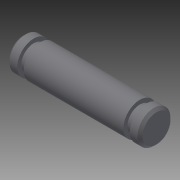
# Autodesk Inventor part: D-9769-clevis_pin
Saved by Autodesk Inventor 2014 (Build 180170000, 170)
## iProperties
Created: 2014-01-19
Part Number: D-9769-clevis_pin
Material: Steel
Catalog Web Link: www.cadenas.de
Description: Pivot Bracket for Original Line Cylinders - Clevis Pin-
Vendor: BIMBA
Document SubType Name: Standard Catalog Part
Designer: Michael
Manufacturer: BIMBA
Density: 7.85 g/cm^3
Appearance: Steel
Mass: 1.44762 g
Surface Area: 2.32572 cm^2
Volume: 0.18441 cm^3
Category: PARTsolutions
Company: BIMBA
PSOL_IDENT_0: {$CADENAS_DATA\23d-libs\bimba\bimba\bimba_imperial\bimba_full_line\original_line_cylinders\accessori
PSOL_IDENT_1: es\clevis_pin.prj},224 {VTYP=3D},{NB=D-9769-clevis_pin},{LINA=D-9769-clevis_pin},{NN=Pivot Bracket f
PSOL_IDENT_2: or Original Line Cylinders - Clevis Pin},{DATE=06.12.2011 07:07:55},{GEOMDATE=06.12.2011 00:00:00},{
PSOL_IDENT_3: VERSION=},{LINEID=30},{LINESUBID=-1},{WBVAR=}  {NB=D-9769-clevis_pin},{LINA=D-9769-clevis_pin},{KT=D
PSOL_IDENT_4: UMMY},{PN=D-9769},{MAT=Zinc-Plated Carbon Steel},{L1=0.46900000},{L2=0.62500000},{L3=0.03000000},{L4=
PSOL_IDENT_5: 0.04800000},{D1=0.15510000},{D2=0.11700000},{CH=0.01200000}
CNS_NN: Pivot Bracket for Original Line Cylinders - Clevis Pin
CNS_NB: D-9769-clevis_pin
CNS_NBSYN: $PN.-clevis_pin
CNS_LINA: D-9769-clevis_pin
CNS_PN: D-9769
CNS_MAT: Zinc-Plated Carbon Steel
CNS_L1: 0.46900000
CNS_L2: 0.62500000
CNS_L3: 0.03000000
CNS_L4: 0.04800000
CNS_D1: 0.15510000
CNS_D2: 0.11700000
CNS_CH: 0.01200000
SUPPLIER: BIMBA
ARTICLENO: D-9769-clevis_pin
BOMINFO: D-9769-clevis_pin
CREATOR: CADENAS GmbH
Title: D-9769-clevis_pin
Author: Cadenas PARTsolutions
Autodesk Inventor part; units mm, degrees
ref_plane "YZ Plane" through (0, 0, 0) normal (1, 0, 0) x (0, 1, 0)
ref_plane "XZ Plane" through (0, 0, 0) normal (0, 1, 0) x (-1, 0, 0)
ref_plane "XY Plane" through (0, 0, 0) normal (0, 0, 1) x (1, 0, 0)
sketch "Sketch_1" plane through (0, 0, 0) normal (0, 0, 1) x (1, 0, 0)
  line L0 (15.875, 0) -> (0, 0)
  line L1 (0, 0) -> (0, 1.665)
  line L2 (0, 1.665) -> (0.3048, 1.9698)
  line L3 (0.3048, 1.9698) -> (1.2192, 1.9698)
  line L4 (1.2192, 1.9698) -> (1.2192, 1.4859)
  line L5 (1.2192, 1.4859) -> (1.9812, 1.4859)
  line L6 (1.9812, 1.4859) -> (1.9812, 1.9698)
  line L7 (1.9812, 1.9698) -> (13.8938, 1.9698)
  line L8 (13.8938, 1.9698) -> (13.8938, 1.4859)
  line L9 (13.8938, 1.4859) -> (14.6558, 1.4859)
  line L10 (14.6558, 1.4859) -> (14.6558, 1.9698)
  line L11 (14.6558, 1.9698) -> (15.5702, 1.9698)
  line L12 (15.5702, 1.9698) -> (15.875, 1.665)
  line L13 (15.875, 1.665) -> (15.875, 0)
  line L14 (15.875, 0) -> (0, 0)
  constraints: 30 end point
revolve "Revolution1" add sketch "Sketch_1" angle 360 about axis through (15.875, 0, 0) along (1, 0, 0)
ref_plane "pin_XY" through (7.9375, 0, 0) normal (1, 0, 0) x (0, 0, -1)
ref_plane "pin_YZ" through (7.9375, 0, 0) normal (0, 0, -1) x (0, 1, 0)
ref_plane "pin_ZX" through (7.9375, 0, 0) normal (0, 1, 0) x (1, 0, 0)
ref_plane "rr1_XY" through (1.6002, 0, 0) normal (1, 0, 0) x (0, 0, -1)
ref_plane "rr1_YZ" through (1.6002, 0, 0) normal (0, 0, -1) x (0, 1, 0)
ref_plane "rr1_ZX" through (1.6002, 0, 0) normal (0, 1, 0) x (1, 0, 0)
ref_plane "rr2_XY" through (14.2748, 0, 0) normal (1, 0, 0) x (0, 0, -1)
ref_plane "rr2_YZ" through (14.2748, 0, 0) normal (0, 0, -1) x (0, 1, 0)
ref_plane "rr2_ZX" through (14.2748, 0, 0) normal (0, 1, 0) x (1, 0, 0)
body "Solid1"
